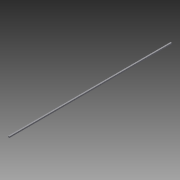
# Autodesk Inventor part: Part3
Saved by Autodesk Inventor 2014 (Build 180170000, 170)
## iProperties
Created: 2014-01-31
Part Number: Part3
Material: Generic
Document SubType Name: Modeling
Designer: JosephLyons
Density: 1 g/cm^3
Appearance: Default
Author: JosephLyons
Autodesk Inventor part; units mm, degrees
ref_plane "YZ Plane" through (0, 0, 0) normal (1, 0, 0) x (0, 1, 0)
ref_plane "XZ Plane" through (0, 0, 0) normal (0, 1, 0) x (-1, 0, 0)
ref_plane "XY Plane" through (0, 0, 0) normal (0, 0, 1) x (1, 0, 0)
sketch "Sketch1" plane through (0, 0, 0) normal (1, 0, 0) x (0, 1, 0)
  line L0 (74.8467, 543.5669) -> (81.1967, 543.5669)
  line L1 (81.1967, 543.5669) -> (81.1967, -281.9331)
  line L2 (81.1967, -281.9331) -> (74.8467, -281.9331)
  line L3 (74.8467, -281.9331) -> (74.8467, 543.5669)
  point P0 (0, 0)
  dimension "d0" = 825.5
  dimension "d1" = 6.35
  constraints: 8 end point, 2 parallel, 1 horizontal, 1 perpendicular
  measures "d0" distance of L0.end L1.end
  measures "d1" distance of L0.start L0.end
extrude "Extrusion1" add sketch "Sketch1" along normal blind 6.35
body "Solid1"
